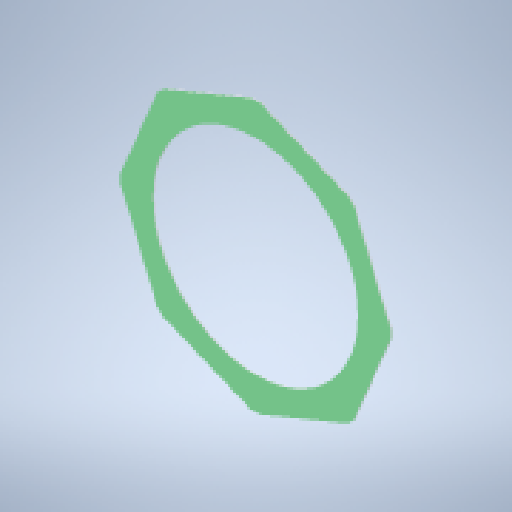
# Autodesk Inventor part: ДМФ 01 29 Барабан сборочный лист
Saved by Autodesk Inventor 2024.2 (Build 282272000, 272)
## iProperties
Created: 2024-04-28
Part Number: ДМФ 01 29 Барабан сборочный лист
Material: Generic
Document SubType Name: Sheet Metal
Designer: admin
Density: 1 g/cm^3
Flat Pattern Width: 54.5449 cm
Flat Pattern Length: 54.5449 cm
Flat Pattern Area: 2975.14 cm^2
Sheet Metal Rule: Default
Sheet Metal Width: 545,449 mm
Sheet Metal Length: 545,449 mm
Sheet Metal Area: 297514,334 mm^2
Appearance: Default
Author: pokla
Autodesk Inventor part; units mm, degrees
ref_plane "YZ Plane" through (0, 0, 0) normal (1, 0, 0) x (0, 1, 0)
ref_plane "XZ Plane" through (0, 0, 0) normal (0, 1, 0) x (-1, 0, 0)
ref_plane "XY Plane" through (0, 0, 0) normal (0, 0, 1) x (1, 0, 0)
sketch "Sketch2" plane through (0, 0, 0) normal (0, 0, 1) x (1, 0, 0)
  line L0 (-195.5512, 195.5512) -> (0, 276.5512)
  line L1 (0, 276.5512) -> (195.5512, 195.5512)
  line L2 (195.5512, 195.5512) -> (276.5512, 0)
  line L3 (276.5512, 0) -> (195.5512, -195.5512)
  line L4 (195.5512, -195.5512) -> (0, -276.5512)
  line L5 (0, -276.5512) -> (-195.5512, -195.5512)
  line L6 (-195.5512, -195.5512) -> (-276.5512, 0)
  line L7 (-276.5512, 0) -> (-195.5512, 195.5512)
  circle A0 centre (0, 0) radius 207.5
  dimension "d23" = 511
  dimension "d26" = 415
  measures "d23" distance between parallel lines of L6 L2
  measures "d26" diameter of A0
extrude "Plate1" add sketch "Sketch2" against normal blind 2
sketch "Sketch5" plane through (0, 0, 0) normal (0, 0, 1) x (1, 0, 0)
  line L0 (0, -276.5512) -> (195.5512, -195.5512) projected
  line L1 (98.6995, -235.6685) -> (97.3929, -235.1273)
  line L2 (97.3929, -235.1273) -> (96.8517, -236.4339)
  line L3 (97.3929, -235.1273) -> (97.7756, -236.0512) construction
  point P0 (0, 0)
  dimension "d30" = 1
  constraints: 6 end point, 3 perpendicular, 2 point on line, 1 midpoint
  measures "d30" distance of L1.end L3.end
chamfer "Chamfer1" distance 10 angle 45 8 edges at (0, 276.5512, -1) (-195.5512, 195.5512, -1) (-276.5512, 0, -1) (-195.5512, -195.5512, -1) (0, -276.5512, -1) (195.5512, -195.5512, -1) (276.5512, 0, -1) (195.5512, 195.5512, -1)
extrude "Extrusion2" cut sketch "Sketch5" along normal through all both and the other way through all
pattern_circular "Circular Pattern2" count 8 over 360 about axis through (0, 0, -10) along (0, 0, 1) of "Extrusion2"
equation "\"d23\" = Барабан_габарит_по_кассетам - 2 * Thickness"
equation "\"d15\" = Thickness"
equation "\"BendRadius\" = Thickness"
equation "\"BendReliefWidth\" = Thickness"
equation "\"BendReliefDepth\" = 0.5 * Thickness"
equation "\"CornerReliefSize\" = 4 * Thickness"
equation "\"MinimumRemnant\" = 2 * Thickness"
equation "\"TransitionRadius\" = BendRadius"
equation "\"JacobiRadiusSize\" = BendRadius"
equation "\"GapSize\" = Thickness"
equation "\"Барабан_габарит_по_кассетам\" = 515"
equation "\"Thickness\" = 2"
body "Solid1"
